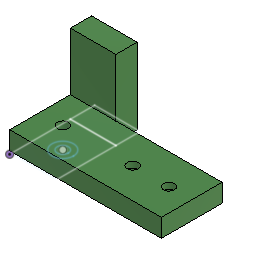
cetus2YEndStop v4 (Autodesk Fusion 360 design; units mm, degrees)
Autodesk Fusion 360 part; units mm, degrees
sketch "Sketch1" plane through (0, 0, 0) normal (0, 0, 1) x (1, 0, 0)
  circle A0 centre (7.5, 10) radius 1.8
  line L0 (0, 0) -> (15, 0)
  line L1 (15, 0) -> (15, 20)
  line L2 (15, 20) -> (0, 20)
  line L3 (0, 20) -> (0, 0)
  circle A1 centre (7.5, 10) radius 3.5
  line L4 (15, 20) -> (0, 20)
  line L5 (0, 20) -> (0, 28)
  line L6 (0, 28) -> (15, 28)
  line L7 (15, 28) -> (15, 20)
  dimension "d3" = 3.6
  dimension "d17" = 15
  dimension "d18" = 20
  dimension "d19" = 10
  dimension "d21" = 7
  dimension "d26" = 15
  dimension "d27" = 8
  constraint horizontal L0
  constraint vertical L1
  constraint horizontal L2
  constraint vertical L3
  constraint coincident L0.start L3.end
  constraint concentric A0 A1
  constraint horizontal L4
  constraint vertical L5
  constraint horizontal L6
  constraint vertical L7
  measures "d3" diameter of A0
  measures "d17" distance of L0.start L0.end
  measures "d18" distance of L0.start L2.end
  measures "d19" distance of A0.centre L2
  measures "d21" diameter of A1
  measures "d26" distance of L1.end L2.end
  measures "d27" distance of L1.end L6.end
extrude "Extrude1" add sketch "Sketch1" along normal blind 7 contours L0 L1 L2 L3 L4 | A1
sketch "Sketch4" plane through (15, 0, 0) normal (1, 0, 0) x (0, 1, 0)
  line L0 (0, 0) -> (20, 0)
  line L1 (20, 0) -> (20, 7)
  line L2 (20, 7) -> (0, 7)
  line L3 (0, 7) -> (0, 0)
extrude "Extrude4" cut sketch "Sketch1" along normal blind 4 contours A1
extrude "Extrude5" add sketch "Sketch1" along normal blind 26 contours L2 L4 L5 L6 L7
extrude "Extrude6" add sketch "Sketch4" along normal blind 35
sketch "Sketch5" plane through (0, 0, 0) normal (0, 0, -1) x (1, 0, 0)
  circle A0 centre (7.5, -10) radius 3.5
  line L0 (50, 0) -> (0, 0)
  line L1 (0, 0) -> (0, -28)
  line L2 (0, -28) -> (15, -28)
  line L3 (15, -28) -> (15, -20)
  line L4 (15, -20) -> (50, -20)
  line L5 (50, -20) -> (50, 0)
  circle A1 centre (42.5, -10) radius 1.8
  circle A2 centre (42.5, -10) radius 3.5
  circle A3 centre (30.5, -10) radius 1.8
  circle A4 centre (30.5, -10) radius 3.5
  point P0 (7.5, -10)
  dimension "d33" = 3.6
  dimension "d34" = 7
  dimension "d35" = 7.5
  dimension "d40" = 3.6
  dimension "d41" = 7
  dimension "d42" = 12
  constraint concentric A1 A2
  constraint concentric A3 A4
  constraint horizontal A1.centre A3.centre
  constraint horizontal A3.centre P0
  measures "d33" diameter of A1
  measures "d34" diameter of A2
  measures "d35" distance of L5 A1.centre
  measures "d40" diameter of A3
  measures "d41" diameter of A4
  measures "d42" distance of A1.centre A3.centre
extrude "Extrude8" cut sketch "Sketch5" against normal through all contours A1 | A3
extrude "Extrude7" cut sketch "Sketch5" against normal blind 5 contours A1 | A2 | A4
chamfer "Chamfer2" distance 1 angle 45 2 faces at (7.4128, 20.4967, 0) (5, 28, 8.6667)
equation "d7 = 7 mm"
equation "d19 = d18 / 2"
equation "d33 = d3"
equation "d34 = d21"
equation "d36 = -d7 + 2 mm"
equation "d40 = d3"
equation "d41 = d21"
